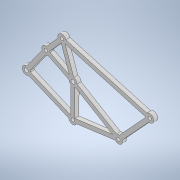
# Autodesk Inventor part: ギア抑え
Saved by Autodesk Inventor 2022.2 (Build 262287030, 287C)
## iProperties
Created: 2022-01-29
Part Number: ギア抑え
Material: Generic
Document SubType Name: Modeling
Designer: acps
Density: 1 g/cm^3
Appearance: Default
Author: acps
Autodesk Inventor part; units mm, degrees
ref_plane "YZ Plane" through (0, 0, 0) normal (1, 0, 0) x (0, 1, 0)
ref_plane "XZ Plane" through (0, 0, 0) normal (0, 1, 0) x (-1, 0, 0)
ref_plane "XY Plane" through (0, 0, 0) normal (0, 0, 1) x (1, 0, 0)
sketch "Sketch2" plane through (0, 0, 0) normal (0, 0, 1) x (1, 0, 0)
  line L0 (46.4683, 30) -> (66.4734, 20) construction
  line L1 (45.7976, 28.6583) -> (65.8027, 18.6583)
  line L2 (67.1441, 21.3417) -> (47.139, 31.3417)
  arc A0 (47.139, 31.3417) -> (45.7976, 28.6583) centre (46.4683, 30) ccw
  arc A1 (65.8027, 18.6583) -> (67.1441, 21.3417) centre (66.4734, 20) ccw
  line L3 (123.045, 25) -> (100, 0) construction
  line L4 (121.9421, 26.0167) -> (98.8971, 1.0167)
  line L5 (101.1029, -1.0167) -> (124.1479, 23.9833)
  arc A2 (124.1479, 23.9833) -> (121.9421, 26.0167) centre (123.045, 25) ccw
  arc A3 (98.8971, 1.0167) -> (101.1029, -1.0167) centre (100, 0) ccw
  line L6 (100, 0) -> (66.299, -4.4994) construction
  line L7 (99.8015, 1.4868) -> (66.1005, -3.0126)
  line L8 (66.4975, -5.9862) -> (100.1985, -1.4868)
  arc A4 (100.1985, -1.4868) -> (99.8015, 1.4868) centre (100, 0) ccw
  arc A5 (66.1005, -3.0126) -> (66.4975, -5.9862) centre (66.299, -4.4994) ccw
  line L9 (32, 10) -> (46.4683, 30) construction
  line L10 (33.2153, 9.1208) -> (47.6836, 29.1208)
  line L11 (45.253, 30.8792) -> (30.7847, 10.8792)
  arc A6 (30.7847, 10.8792) -> (33.2153, 9.1208) centre (32, 10) ccw
  arc A7 (47.6836, 29.1208) -> (45.253, 30.8792) centre (46.4683, 30) ccw
  line L12 (32, 10) -> (66.299, -4.4994) construction
  line L13 (31.4159, 8.6184) -> (65.715, -5.881)
  line L14 (66.8831, -3.1178) -> (32.5841, 11.3816)
  arc A8 (32.5841, 11.3816) -> (31.4159, 8.6184) centre (32, 10) ccw
  arc A9 (65.715, -5.881) -> (66.8831, -3.1178) centre (66.299, -4.4994) ccw
  line L15 (46.4683, 30) -> (58.3063, 43.4) construction
  line L16 (47.5924, 29.0069) -> (59.4305, 42.4069)
  line L17 (57.1822, 44.3931) -> (45.3441, 30.9931)
  arc A10 (45.3441, 30.9931) -> (47.5924, 29.0069) centre (46.4683, 30) ccw
  arc A11 (59.4305, 42.4069) -> (57.1822, 44.3931) centre (58.3063, 43.4) ccw
  line L18 (58.3063, 43.4) -> (66.4734, 20) construction
  line L19 (56.8901, 42.9057) -> (65.0572, 19.5057)
  line L20 (67.8896, 20.4943) -> (59.7225, 43.8943)
  arc A12 (59.7225, 43.8943) -> (56.8901, 42.9057) centre (58.3063, 43.4) ccw
  arc A13 (65.0572, 19.5057) -> (67.8896, 20.4943) centre (66.4734, 20) ccw
  line L21 (66.4734, 20) -> (66.299, -4.4994) construction
  line L22 (64.9735, 20.0107) -> (64.7991, -4.4887)
  line L23 (67.799, -4.5101) -> (67.9734, 19.9893)
  arc A14 (67.9734, 19.9893) -> (64.9735, 20.0107) centre (66.4734, 20) ccw
  arc A15 (64.7991, -4.4887) -> (67.799, -4.5101) centre (66.299, -4.4994) ccw
  line L24 (66.4734, 20) -> (100, 0) construction
  line L25 (65.705, 18.7118) -> (99.2315, -1.2882)
  line L26 (100.7685, 1.2882) -> (67.2419, 21.2882)
  arc A16 (67.2419, 21.2882) -> (65.705, 18.7118) centre (66.4734, 20) ccw
  arc A17 (99.2315, -1.2882) -> (100.7685, 1.2882) centre (100, 0) ccw
  line L27 (58.3063, 43.4) -> (123.045, 25) construction
  line L28 (57.8962, 41.9571) -> (122.6349, 23.5571)
  line L29 (123.4551, 26.4429) -> (58.7164, 44.8429)
  arc A18 (58.7164, 44.8429) -> (57.8962, 41.9571) centre (58.3063, 43.4) ccw
  arc A19 (122.6349, 23.5571) -> (123.4551, 26.4429) centre (123.045, 25) ccw
  circle A20 centre (46.4683, 30) radius 3
  circle A21 centre (58.3063, 43.4) radius 3
  circle A22 centre (123.045, 25) radius 3
  circle A23 centre (66.4734, 20) radius 3
  circle A24 centre (100, 0) radius 3
  circle A25 centre (66.299, -4.4994) radius 3
  circle A26 centre (32, 10) radius 3
  circle A27 centre (46.4683, 30) radius 1.25
  circle A28 centre (58.3063, 43.4) radius 1.25
  circle A29 centre (123.045, 25) radius 1.25
  circle A30 centre (100, 0) radius 1.25
  circle A31 centre (66.299, -4.4994) radius 1.25
  circle A32 centre (32, 10) radius 1.5
  point P0 (0, 0)
  point P1 (63.4788, 19.8199)
  point P2 (64.955, 17.4127)
  point P3 (64.8119, -2.686)
  point P4 (47.0701, 27.061)
  point P5 (48.1215, 27.4966)
  point P6 (63.8273, 22.9997)
  point P7 (49.4629, 30.1801)
  point P8 (49.3126, 30.954)
  point P9 (57.7343, 40.4869)
  point P10 (63.8353, 23.0067)
  point P11 (69.4731, 19.9572)
  point P12 (67.0335, 22.9473)
  point P13 (60.6742, 41.1676)
  point P14 (120.1358, 24.2674)
  point P15 (120.1812, 24.1064)
  point P16 (100.658, 2.927)
  point P17 (98.5372, 2.6192)
  point P18 (95.5346, 0.9171)
  point P19 (67.8113, -2.7842)
  point P20 (67.9547, 17.3697)
  point P21 (47.0643, 32.9402)
  point P22 (44.2209, 28.0127)
  point P23 (66.0689, -5.9816)
  point P24 (66.4975, -5.9862)
  point P25 (97.6233, -1.8306)
  point P26 (102.8638, 0.8936)
  point P27 (122.387, 22.073)
  point P28 (120.956, 27.1531)
  point P29 (61.2155, 44.1326)
  point P30 (55.462, 42.446)
  point P31 (99.2315, -1.2882)
  point P32 (99.2644, 1.4151)
  point P33 (100.7685, 1.2882)
  point P34 (65.8027, 18.6583)
  point P35 (65.705, 18.7118)
  point P36 (67.1441, 21.3417)
  point P37 (45.3441, 30.9931)
  point P38 (47.139, 31.3417)
  point P39 (47.7709, 29.2089)
  point P40 (56.4708, 25)
  point P41 (111.5225, 12.5)
  point P42 (83.1495, -2.2497)
  point P43 (39.2341, 20)
  point P44 (49.1495, 2.7503)
  point P45 (52.3873, 36.7)
  point P46 (62.3899, 31.7)
  point P47 (66.3862, 7.7503)
  point P48 (83.2367, 10)
  point P49 (90.6757, 34.2)
  point P50 (49.4629, 30.1801)
  point P51 (49.3126, 30.954)
  point P52 (57.7343, 40.4869)
  point P53 (63.8399, 22.9934)
  point P54 (48.1215, 27.4966)
  point P55 (63.4788, 19.8199)
  point P56 (64.955, 17.4127)
  point P57 (64.815, -2.2435)
  point P58 (34.9771, 10.37)
  point P59 (34.7381, 11.2258)
  point P60 (46.1608, 27.0158)
  point P61 (60.6742, 41.1676)
  point P62 (120.1358, 24.2674)
  point P63 (120.1812, 24.1064)
  point P64 (100.658, 2.927)
  point P65 (98.5372, 2.6192)
  point P66 (69.4731, 19.9572)
  point P67 (67.0335, 22.9473)
  point P68 (67.9547, 17.3697)
  point P69 (95.5346, 0.9171)
  point P70 (67.8113, -2.7842)
  point P71 (34.32, 10.6478)
  point P72 (122.387, 22.073)
  point P73 (120.956, 27.1531)
  point P74 (61.2155, 44.1326)
  point P75 (55.462, 42.446)
  point P76 (47.0643, 32.9402)
  point P77 (43.7302, 28.7742)
  point P78 (32.3075, 12.9842)
  point P79 (33.809, 7.6068)
  point P80 (63.3219, -4.8694)
  point P81 (69.0728, -5.6424)
  point P82 (97.6233, -1.8306)
  point P83 (102.8638, 0.8936)
  dimension "d53" = 3
  dimension "d54" = 3
  dimension "d55" = 3
  dimension "d56" = 3
  dimension "d57" = 3
  dimension "d58" = 3
  dimension "d59" = 3
  dimension "d60" = 3
  dimension "d61" = 3
  dimension "d62" = 3
  dimension "d63" = 6
  dimension "d64" = 6
  dimension "d65" = 6
  dimension "d66" = 6
  dimension "d67" = 6
  dimension "d68" = 6
  dimension "d69" = 6
  dimension "d70" = 2.5
  dimension "d71" = 2.5
  dimension "d72" = 2.5
  dimension "d73" = 2.5
  dimension "d74" = 2.5
  dimension "d76" = 3
  constraints: 80 end point, 40 point on circle, 40 tangent, 33 centre point, 17 coincident, 10 midpoint, 10 parallel, 6 concentric, 3 other
  measures "d53" diameter of A1
  measures "d54" diameter of A3
  measures "d55" diameter of A5
  measures "d56" diameter of A7
  measures "d57" diameter of A9
  measures "d58" diameter of A11
  measures "d59" diameter of A13
  measures "d60" diameter of A15
  measures "d61" diameter of A17
  measures "d62" diameter of A19
  measures "d63" diameter of A20
  measures "d64" diameter of A21
  measures "d65" diameter of A22
  measures "d66" diameter of A23
  measures "d67" diameter of A24
  measures "d68" diameter of A25
  measures "d69" diameter of A26
  measures "d70" diameter of A27
  measures "d71" diameter of A28
  measures "d72" diameter of A29
  measures "d73" diameter of A30
  measures "d74" diameter of A31
  measures "d76" diameter of A32
extrude "Extrusion1" add sketch "Sketch2" against normal blind 3 contours A10 L16 L10 L1 | L1 L10 A20 L11 A0 | A0 A7 L10 L16 A10 | L10 L16 L2 A20 L1 | L1 A20 L10 | L11 A20 L17 A0 | A20 L2 L19 A23 L1 | L10 A26 L11 A20 | L10 A7 L2 L16 | L17 A20 L16 L2 A0 | A23 L19 L22 L1 | L1 L22 A23 | A26 L14 L10 | L10 L14 A8 L11 A26 | L16 A20 L2 | L17 A21 L16 A20 | L11 A6 L13 A26 | L22 L19 A13 L1 | L1 L25 A23 L22 | A23 L2 A14 L22 L19 | L19 L2 A23 | A23 L25 L23 A25 L22 | L14 A26 L13 A6 L10 | L10 A32 L14 | L14 A25 L13 A26 | A21 L29 A11 L17 | L17 A12 L19 L16 A21 | L1 A1 L23 A23 L25 | L22 A16 L19 | L19 A21 L28 L20 A23 L2 | A23 L20 L26 A1 L2 | A25 L23 L7 L14 L22 | A23 L23 L25 | L14 L22 A5 L13 A25 | A11 L16 L28 A18 A12 | A21 L20 A11 L29 | L29 A22 L28 L20 A21 | L13 A5 L8 A25 | L19 L16 L28 A21 | A23 L26 L20 | L14 L7 A5 L22 | L23 A23 L26 A24 L7 L25 | L23 A1 L20 L26 A23 | L19 A18 L28 L16 | A22 L5 A2 L29 | L29 A2 L4 L28 A22 | A5 L7 L14 A9 | A25 L7 L25 A24 L8 | L8 A9 L23 L7 A25 | A21 L20 L28 | L28 L16 A11 L20 A21 | L26 L20 A1 | L7 L23 A9 L14 | L7 A24 L25 | A2 A19 L28 L4 | L28 L4 A22 | A24 L25 A3 L8 | L8 A3 L5 A24 | A24 L26 L4 L7 | L7 L4 A3 L25 A24 | A24 L4 L26 | L5 A22 L4 L28 A19 | L5 A24 L4 A22 | A3 L4 L7 A4 | L4 L26 A4 L7 | L4 A24 L5 A4 L26
body "Solid1"
